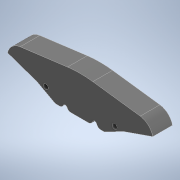
# Autodesk Inventor part: bumper
Saved by Autodesk Inventor 2022 (Build 260153000, 153)
## iProperties
Created: 2022-02-22
Part Number: bumper
Material: Polystyrene, Expanded
Document SubType Name: Modeling
Designer: hugof
Density: 0.05 g/cm^3
Appearance: Gray
Author: hugof
Autodesk Inventor part; units mm, degrees
ref_plane "YZ Plane" through (0, 0, 0) normal (1, 0, 0) x (0, 1, 0)
ref_plane "XZ Plane" through (0, 0, 0) normal (0, 1, 0) x (-1, 0, 0)
ref_plane "XY Plane" through (0, 0, 0) normal (0, 0, 1) x (1, 0, 0)
sketch "Sketch1" plane through (0, 0, 0) normal (0, 0, 1) x (1, 0, 0)
  line L0 (0, 0) -> (-48.9676, 0)
  line L1 (-147.5, 0) -> (-147.5, 20.4375)
  line L2 (-147.5, 40) -> (-73.75, 40)
  line L3 (0, 40) -> (0, 30.4375)
  line L4 (-108.75, 10) -> (-38.75, 10)
  line L5 (-108.75, 10) -> (-117.5, 10)
  line L6 (-38.75, 10) -> (-30, 10)
  line L7 (-98.9676, 0) -> (-92.4032, 0)
  line L8 (-147.5, 0) -> (-98.9676, 0)
  line L9 (-48.9676, 0) -> (0, 0)
  line L10 (-147.5, 10) -> (-117.5, 10)
  line L11 (0, 10) -> (-30, 10)
  line L12 (-98.9676, 0) -> (-117.5, 10)
  line L13 (-48.9676, 0) -> (-30, 10)
  line L14 (-117.5, 10) -> (-147.5, 10)
  line L15 (-30, 10) -> (0, 10)
  circle A0 centre (-108.75, 10) radius 2.5
  circle A1 centre (-38.75, 10) radius 2.5
  line L16 (-147.5, 10) -> (-147.5, 20.4375)
  line L17 (-117.5, 10) -> (-147.5, 20.4375)
  line L18 (0, 10) -> (0, 20.4375)
  line L19 (0, 20.4375) -> (-147.5, 20.4375)
  line L20 (-30, 10) -> (0, 20.4375)
  line L21 (-147.5, 20.4375) -> (-147.5, 30.4375)
  line L22 (-147.5, 30.4375) -> (-73.75, 40)
  line L23 (0, 20.4375) -> (0, 30.4375)
  line L24 (-73.75, 40) -> (0, 30.4375)
  line L25 (0, 20.4375) -> (0, 0)
  line L26 (0, 30.4375) -> (0, 20.4375)
  line L27 (-147.5, 30.4375) -> (-147.5, 40)
  line L28 (-147.5, 20.4375) -> (-147.5, 30.4375)
  line L29 (-73.75, 40) -> (0, 40)
  line L30 (-88.7871, 0) -> (-58.7871, 0)
  line L31 (-88.7575, 0) -> (-58.7871, 0)
  line L32 (-88.7575, 0) -> (-88.7575, 6.2461)
  line L33 (-58.7871, 0) -> (-58.7871, 7.0063)
  line L34 (-58.7871, 7.0063) -> (-62.8766, 0)
  line L35 (-58.7871, 7.0063) -> (-55.532, 0)
  line L36 (-88.7575, 6.2461) -> (-85.8556, 0)
  line L37 (-88.7575, 6.2461) -> (-92.4032, 0)
  line L38 (-58.7871, 0) -> (-55.532, 0)
  line L39 (-92.4032, 0) -> (-147.5, 0)
  line L40 (-48.9676, 0) -> (-55.532, 0)
  line L41 (-55.532, 0) -> (-92.4032, 0)
  line L42 (-92.4032, 0) -> (-88.7575, 0)
  line L43 (-55.532, 0) -> (-48.9676, 0)
  point P0 (-73.75, 0)
  point P1 (-85.8556, 0)
  dimension "d0" = 147.5
  dimension "d1" = 40
  dimension "d2" = 70
  dimension "d3" = 10
  dimension "d4" = 50
  dimension "d5" = 30
  dimension "d6" = 30
  dimension "d7" = 5
  dimension "d8" = 5
  dimension "d9" = 10
  dimension "d10" = 30
  constraints: 88 end point, 19 parallel, 19 perpendicular, 12 point on line, 8 horizontal, 4 collinear, 3 equal length, 2 centre point, 2 coincident, 2 vertical
  measures "d0" distance of L2.start L3.start
  measures "d1" distance of L1.start L2.start
  measures "d2" distance of L4.start L4.end
  measures "d3" distance from line of L4 point (-73.75, 0)
  measures "d4" distance of L0.end L7.start
  measures "d5" distance of L10.start L5.end
  measures "d6" distance of L11.start L6.end
  measures "d7" diameter of A0
  measures "d8" diameter of A1
  measures "d9" distance of L18.end L3.end
  measures "d10" distance of L30.start L30.end
extrude "Extrusion2" add sketch "Sketch1" along normal blind 20 contours L40 L35 L34 L30 L36 L37 L7 L12 L5 A0 L4 A1 L6 L13 | L6 A1 L4 A0 L5 L17 L19 L20 | L19 L21 L22 L24 L23
fillet "Fillet5" radius 100 1 edges at (-73.75, 40, 10)
fillet "Fillet6" radius 15 2 edges at (0, 30.4375, 10) (-147.5, 30.4375, 10)
fillet "Fillet7" radius 10 2 edges at (-117.5, 10, 10) (-30, 10, 10)
fillet "Fillet8" radius 4 6 edges at (-98.9676, 0, 10) (-92.4032, 0, 10) (-55.532, 0, 10) (-48.9676, 0, 10) (-85.8556, 0, 10) (-62.8766, 0, 10)
fillet "Fillet9" radius 2 2 edges at (-88.7575, 6.2461, 10) (-58.7871, 7.0063, 10)
body "Solid2"
